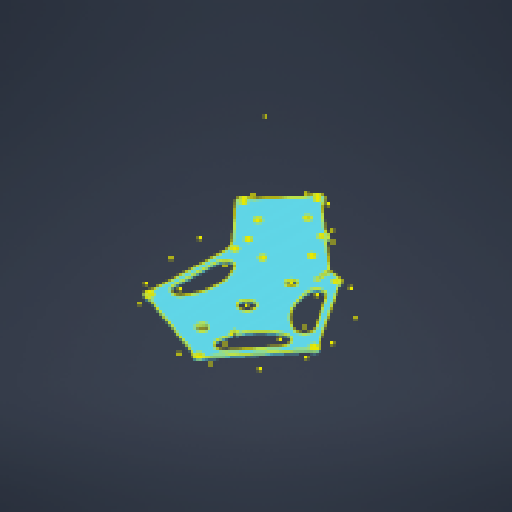
# Autodesk Inventor part: femur_motor_steel
Saved by Autodesk Inventor 2026 (Build 300175000, 175)
## iProperties
Created: 2026-04-24
Part Number: femur_motor_steel
Material: Сталь
Document SubType Name: Modeling
Designer: user
Density: 7.85 g/cm^3
Appearance: Серо-синий
Author: user
Autodesk Inventor part; units mm, degrees
ref_plane "YZ Plane" through (0, 0, 0) normal (1, 0, 0) x (0, 1, 0)
ref_plane "XZ Plane" through (0, 0, 0) normal (0, 1, 0) x (-1, 0, 0)
ref_plane "XY Plane" through (0, 0, 0) normal (0, 0, 1) x (1, 0, 0)
sketch "Эскиз1" plane through (0, 0, 0) normal (0, 1, 0) x (-1, 0, 0)
  circle A0 centre (-102.5556, 225.6292) radius 3.05
  circle A1 centre (-183.8617, 259.7302) radius 3.05
  circle A2 centre (-241.4187, 192.9413) radius 3.05
  circle A3 centre (-195.6847, 117.5625) radius 3.05
  circle A4 centre (-109.8626, 137.7647) radius 3.05
  line L0 (-177.5294, 108.3895) -> (-150.4825, 84.7228) projected
  arc A5 (-148.7964, 81.4219) -> (-142.475, 75.8905) centre (-142.7225, 81.9854) ccw projected
  line L1 (-138.9795, 74.6574) -> (-112.854, 51.7971) projected
  arc A6 (-111.168, 48.4962) -> (-98.9991, 49.3073) centre (-105.0941, 49.0597) ccw projected
  line L2 (-97.7661, 52.8028) -> (-70.8888, 83.5189) projected
  arc A7 (-67.5879, 85.2049) -> (-63.3144, 94.9954) centre (-68.1514, 91.2788) ccw projected
  line L3 (-63.3144, 94.9954) -> (-108.3131, 153.5599) projected
  arc A8 (-154.5301, 238.9315) -> (-170.0329, 240.2208) centre (-162.9261, 231.8247) ccw projected
  line L4 (-186.8375, 143.9878) -> (-185.285, 127.1516) projected
  arc A9 (-185.285, 127.1516) -> (-183.1128, 124.9467) centre (-183.2964, 126.9383) ccw projected
  line L5 (-183.1128, 124.9467) -> (-179.0904, 125.3176) projected
  line L6 (-179.0904, 125.3176) -> (-177.5294, 108.3895) projected
  circle A10 centre (-117.9158, 72.371) radius 3.05 projected
  circle A11 centre (-155.5442, 105.2966) radius 3.05 projected
  circle A12 centre (-130.5866, 133.819) radius 3.05 projected
  circle A13 centre (-105.7799, 124.2045) radius 3.05 projected
  circle A14 centre (-92.9581, 100.8933) radius 3.05 projected
  circle A15 centre (-162.9261, 231.8247) radius 5.05 projected
  circle A16 centre (-121.5775, 182.975) radius 5.05 projected
  circle A17 centre (-105.0941, 49.0597) radius 3.05 projected
  circle A18 centre (-142.7225, 81.9854) radius 3.05 projected
  circle A19 centre (-68.1514, 91.2788) radius 3.05 projected
  line L7 (-182.2769, 125.0238) -> (-180.8753, 109.8244)
  arc A20 (-179.9058, 262.7882) -> (-188.7663, 260.7024) centre (-183.8617, 259.7302) ccw
  arc A21 (-98.4249, 222.8119) -> (-103.1466, 230.5942) centre (-102.5556, 225.6292) ccw
  arc A22 (-200.6825, 117.4137) -> (-196.2371, 112.5931) centre (-195.6847, 117.5625) ccw
  arc A23 (-243.1045, 197.6485) -> (-243.8589, 188.5772) centre (-241.4187, 192.9413) ccw
  line L8 (-180.8753, 109.8244) -> (-196.5681, 112.6411)
  circle A24 centre (-166.6767, 186.7256) radius 85 construction
  line L9 (-99.8729, 142.5753) -> (-63.3144, 94.9954)
  arc A25 (-104.963, 159.8791) -> (-99.8729, 142.5753) centre (-80.049, 157.8072) ccw
  line L10 (-196.2294, 112.5804) -> (-196.2371, 112.5931)
  line L11 (-202.1286, 122.3034) -> (-240.1899, 185.0362)
  line L12 (-100.129, 218.0061) -> (-104.963, 159.8791)
  line L13 (-175.8619, 259.6823) -> (-108.1962, 231.3023)
  line L14 (-77.9802, 218.6293) -> (-73.529, 216.7624)
  arc A26 (-98.4249, 222.8119) -> (-100.129, 218.0061) centre (-90.1634, 217.1773) ccw
  arc A27 (-108.1962, 231.3023) -> (-103.1466, 230.5942) centre (-104.3284, 240.5241) ccw
  arc A28 (-179.9058, 262.7882) -> (-175.8619, 259.6823) centre (-171.9941, 268.9041) ccw
  arc A29 (-191.0002, 256.1188) -> (-188.7663, 260.7024) centre (-198.5754, 262.6469) ccw
  arc A30 (-243.1045, 197.6485) -> (-238.901, 200.5348) centre (-246.4763, 207.0629) ccw
  arc A31 (-240.1899, 185.0362) -> (-243.8589, 188.5772) centre (-248.7394, 179.8491) ccw
  arc A32 (-200.6825, 117.4137) -> (-202.1286, 122.3034) centre (-210.6781, 117.1163) ccw
  arc A33 (-148.7964, 81.4219) -> (-150.4825, 84.7228) centre (-153.775, 80.9599) ccw projected
  arc A34 (-138.9795, 74.6574) -> (-142.475, 75.8905) centre (-142.272, 70.8946) ccw projected
  arc A35 (-111.168, 48.4962) -> (-112.854, 51.7971) centre (-116.1466, 48.0342) ccw projected
  arc A36 (-97.7661, 52.8028) -> (-98.9991, 49.3073) centre (-94.0032, 49.5102) ccw projected
  arc A37 (-67.5879, 85.2049) -> (-70.8888, 83.5189) centre (-67.1259, 80.2263) ccw projected
  arc A38 (-173.2989, 194.5492) -> (-160.0544, 178.902) centre (-166.6767, 186.7256) ccw projected
  arc A39 (-111.4672, 178.6413) -> (-108.3131, 153.5599) centre (-88.4892, 168.7918) ccw projected
  arc A40 (-111.4672, 178.6413) -> (-113.1815, 190.0818) centre (-121.5775, 182.975) ccw projected
  line L15 (-113.1815, 190.0818) -> (-127.2335, 206.6831) projected
  line L16 (-127.2335, 206.6831) -> (-160.0544, 178.902) projected
  line L17 (-173.2989, 194.5492) -> (-140.478, 222.3303) projected
  line L18 (-140.478, 222.3303) -> (-154.5301, 238.9315) projected
  line L19 (-170.0329, 240.2208) -> (-188.2631, 224.7899) projected
  arc A41 (-218.8826, 198.8722) -> (-220.1719, 183.3693) centre (-211.7758, 190.4761) ccw projected
  line L20 (-220.1719, 183.3693) -> (-186.8375, 143.9878) projected
  circle A42 centre (-170.4272, 141.6264) radius 5.05 projected
  circle A43 centre (-211.7758, 190.4761) radius 5.05 projected
  arc A44 (-154.7115, 183.4245) -> (-167.956, 199.0717) centre (-161.3337, 191.2481) ccw
  line L21 (-220.9265, 180.3759) -> (-221.3765, 181.0768)
  line L22 (-190.4765, 248.7938) -> (-191.1373, 255.9597)
  line L23 (-193.663, 248.4999) -> (-194.0403, 252.5911)
  line L24 (-190.4765, 248.7938) -> (-193.663, 248.4999)
  line L25 (-238.901, 200.5348) -> (-194.0403, 252.5911)
  line L26 (-191.1373, 255.9597) -> (-191.0002, 256.1188)
  line L27 (-188.2631, 224.7899) -> (-187.4464, 215.9332) projected
  line L28 (-187.4464, 215.9332) -> (-190.6328, 215.6393) projected
  line L29 (-190.6328, 215.6393) -> (-191.244, 222.2668) projected
  line L30 (-191.244, 222.2668) -> (-218.8826, 198.8722) projected
  point P0 (0, 0)
  point P1 (-98.7723, 141.1427)
  point P2 (-176.2905, 107.3053)
  point P3 (-200.3475, 119.3677)
  point P4 (-241.9711, 187.9719)
  point P5 (-241.1427, 197.9337)
  point P6 (-179.0284, 261.0104)
  point P7 (-188.7586, 258.72)
  point P8 (-99.8445, 221.4281)
  point P9 (-105.0296, 229.9742)
  point P10 (-99.8729, 142.5753)
  point P11 (-236.553, 192.5367)
  dimension "d5" = 6.1
  dimension "d8" = 360
  dimension "d13" = 3.2
  dimension "d16" = 10
  dimension "d26" = 170
  dimension "d31" = 25
  dimension "d32" = 10
  dimension "d33" = 10
  dimension "d34" = 10
  dimension "d35" = 10
  dimension "d36" = 7
  dimension "d37" = 75
  dimension "d46" = 124
  constraints: 36 tangent, 34 point on circle, 28 end point, 19 centre point, 13 point on line, 6 coincident, 6 equal radius, 2 collinear, 1 parallel, 1 perpendicular, 12 other
  measures "d5" diameter of A0
  measures "d13" distance between parallel lines of L6 L7
  measures "d16" diameter of A20
  measures "d26" diameter of A24
  measures "d31" radius of A25
  measures "d32" radius of A26
  measures "d33" radius of A30
  measures "d34" radius of A31
  measures "d35" radius of A32
  measures "d36" distance of A44.centre point (-166.677, 186.726)
  measures "d37" distance of A3.centre point (-166.677, 186.726)
  measures "d46" distance from line of L22.start L5
extrude "Выдавливание1" add sketch "Эскиз1" along normal blind 3 contours L6 L5 A9 L4 L20 A41 L30 L29 L28 L27 L19 A8 L18 L17 A38 L16 L15 A40 A39 L3 A7 A37 L2 A36 A6 A35 L1 A34 A5 A33 L0 | L7 L8 L10 A22 A32 L11 A31 A23 A30 L25 L23 L24 L22 L26 A29 A20 A28 L13 A27 A21 A26 L12 A25 L3 A39 A40 L15 L16 A44 L17 L18 A8 L19 L27 L28 L29 L30 A41 L20 L4 A9 L5 | L8 A22 L10
sketch "Эскиз2" plane through (0, 3, 0) normal (0, 1, 0) x (1, 0, 0)
  line L0 (63.3144, -94.9954) -> (99.8729, -142.5753) projected
  arc A0 (104.963, -159.8791) -> (99.8729, -142.5753) centre (80.049, -157.8072) ccw projected
  line L1 (104.963, -159.8791) -> (100.129, -218.0061) projected
  arc A1 (98.4249, -222.8119) -> (100.129, -218.0061) centre (90.1634, -217.1773) ccw projected
  arc A2 (98.4249, -222.8119) -> (103.1466, -230.5942) centre (102.5556, -225.6292) ccw projected
  arc A3 (108.1962, -231.3023) -> (103.1466, -230.5942) centre (104.3284, -240.5241) ccw projected
  line L2 (108.1962, -231.3023) -> (175.8619, -259.6823) projected
  arc A4 (179.9058, -262.7882) -> (175.8619, -259.6823) centre (171.9941, -268.9041) ccw projected
  arc A5 (179.9058, -262.7882) -> (188.7663, -260.7024) centre (183.8617, -259.7302) ccw projected
  arc A6 (191.0002, -256.1188) -> (188.7663, -260.7024) centre (198.5754, -262.6469) ccw projected
  line L3 (194.0403, -252.5911) -> (238.901, -200.5348) projected
  arc A7 (243.1045, -197.6485) -> (238.901, -200.5348) centre (246.4763, -207.0629) ccw projected
  arc A8 (243.1045, -197.6485) -> (243.8589, -188.5772) centre (241.4187, -192.9413) ccw projected
  arc A9 (240.1899, -185.0362) -> (243.8589, -188.5772) centre (248.7394, -179.8491) ccw projected
  line L4 (240.1899, -185.0362) -> (202.1286, -122.3034) projected
  arc A10 (200.6825, -117.4137) -> (202.1286, -122.3034) centre (210.6781, -117.1163) ccw projected
  arc A11 (200.6825, -117.4137) -> (196.5681, -112.6411) centre (195.6847, -117.5625) ccw projected
  line L5 (196.5681, -112.6411) -> (180.8753, -109.8244) projected
  line L6 (180.8753, -109.8244) -> (182.2769, -125.0238) projected
  line L7 (182.2769, -125.0238) -> (179.0904, -125.3176) projected
  line L8 (179.0904, -125.3176) -> (177.5294, -108.3895) projected
  line L9 (177.5294, -108.3895) -> (150.4825, -84.7228) projected
  arc A12 (148.7964, -81.4219) -> (150.4825, -84.7228) centre (153.775, -80.9599) ccw projected
  arc A13 (148.7964, -81.4219) -> (142.475, -75.8905) centre (142.7225, -81.9854) ccw projected
  arc A14 (138.9795, -74.6574) -> (142.475, -75.8905) centre (142.272, -70.8946) ccw projected
  line L10 (138.9795, -74.6574) -> (112.854, -51.7971) projected
  arc A15 (111.168, -48.4962) -> (112.854, -51.7971) centre (116.1466, -48.0342) ccw projected
  arc A16 (111.168, -48.4962) -> (98.9991, -49.3073) centre (105.0941, -49.0597) ccw projected
  arc A17 (97.7661, -52.8028) -> (98.9991, -49.3073) centre (94.0032, -49.5102) ccw projected
  line L11 (97.7661, -52.8028) -> (70.8888, -83.5189) projected
  arc A18 (67.5879, -85.2049) -> (70.8888, -83.5189) centre (67.1259, -80.2263) ccw projected
  arc A19 (67.5879, -85.2049) -> (63.3144, -94.9954) centre (68.1514, -91.2788) ccw projected
  circle A20 centre (109.8626, -137.7647) radius 3.05 projected
  circle A21 centre (117.9158, -72.371) radius 3.05 projected
  circle A22 centre (155.5442, -105.2966) radius 3.05 projected
  circle A23 centre (105.7799, -124.2045) radius 3.05 projected
  circle A24 centre (92.9581, -100.8933) radius 3.05 projected
  circle A25 centre (162.9261, -231.8247) radius 5.05 projected
  circle A26 centre (105.0941, -49.0597) radius 3.05 projected
  circle A27 centre (142.7225, -81.9854) radius 3.05 projected
  circle A28 centre (68.1514, -91.2788) radius 3.05 projected
  circle A29 centre (130.5866, -133.819) radius 3.05 projected
  circle A30 centre (195.6847, -117.5625) radius 3.05 projected
  circle A31 centre (241.4187, -192.9413) radius 3.05 projected
  circle A32 centre (183.8617, -259.7302) radius 3.05 projected
  circle A33 centre (102.5556, -225.6292) radius 3.05 projected
  line L12 (191.0002, -256.1188) -> (191.1373, -255.9597) projected
  line L13 (191.1373, -255.9597) -> (190.4765, -248.7938) projected
  line L14 (190.4765, -248.7938) -> (193.663, -248.4999) projected
  line L15 (193.663, -248.4999) -> (194.0403, -252.5911) projected
  point P0 (0, 0)
equation "\"d5\" = d_main_screw_holes"
equation "\"d2\" = thickness_steel"
equation "\"tolerance_plazma\" = 0.1"
equation "\"thickness_steel\" = 3"
equation "\"d_main_screw_holes\" = 6.1"
equation "\"thickness_profile_tibea\" = 3"
equation "\"hight_shaft_shift\" = 37"
equation "\"thickness_profile_femur\" = 3"
equation "\"width_shaft_shift\" = 35"
equation "\"width_flattened_surface\" = 12"
equation "\"d22\" = d_main_screw_holes"
equation "\"d23\" = d_main_screw_holes"
equation "\"d25\" = d_main_screw_holes"
